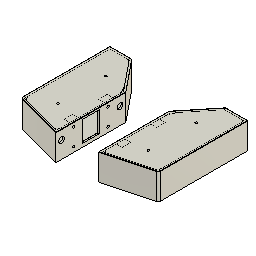
2_Assembly_Chassis v11 (Autodesk Fusion 360 archive; units mm, degrees)
design "Back Extention"
Autodesk Fusion 360 part; units mm, degrees
(part 1 of 2)
sketch "Sketch1" plane through (0, 0, 0) normal (0, 0, 1) x (1, 0, 0)
  line L0 (0, 0) -> (0, 121.8)
  line L1 (0, 0) -> (78.294095, 20.97884)
  line L2 (82, 25.808469) -> (82, 176.135475)
  line L3 (82, 176.135475) -> (44, 176.135475)
  line L4 (44, 176.135475) -> (0, 121.8)
  arc A0 (78.294095, 20.97884) -> (82, 25.808469) centre (77, 25.808469) ccw
  line L5 (3, 3.909676) -> (77.517638, 23.876617)
  arc A1 (77.517638, 23.876617) -> (79, 25.808469) centre (77, 25.808469) ccw
  line L6 (79, 25.808469) -> (79, 173.135475)
  line L7 (79, 173.135475) -> (45.430927, 173.135475)
  line L8 (45.430927, 173.135475) -> (3, 120.737644)
  line L9 (3, 3.909676) -> (3, 120.737644)
  line L10 (3, 91.254041) -> (79, 91.254041) construction
  line L11 (41, 167.663736) -> (41, 14.091745) construction
  circle A2 centre (41, 128.135475) radius 5
  circle A3 centre (41, 45) radius 5
  dimension "d3" = 121.8
  dimension "d4" = 75
  dimension "d5" = 141
  dimension "d6" = 82
  dimension "d7" = 75
  dimension "d8" = 38
  dimension "d9" = 5
  dimension "d64" = -3
  dimension "d86" = 10
  dimension "d87" = 45
  dimension "d88" = 10
  dimension "d89" = 45
  constraint coincident L0.start L1.start
  constraint vertical L0
  constraint parallel L0 L2
  constraint perpendicular L0 L3
  constraint tangent L2 A0
  constraint tangent L1 A0
  constraint perpendicular L6 L10
  constraint perpendicular L10 L11
  constraint coincident L11 A3.centre
  measures "d3" distance of L0.start L0.end
  measures "d4" angle of L0 L1
  measures "d5" angle of L0 L4
  measures "d6" distance of L0 L2
  measures "d7" angle of L0 L1
  measures "d9" radius of A0
  measures "d86" diameter of A2
  measures "d88" diameter of A3
  measures "d89" vertical distance of L0.start A3.centre
extrude "Extrude7" add sketch "Sketch1" along normal blind 3 contours L5 A1 L6 L7 L8 L9 | A2 | A3 picked at (67.925955, 108.535214) picked at (43.631771, 126.680026) picked at (42.542117, 43.337994) makes body 1
extrude "Extrude13" add sketch "Sketch1" along normal blind 45 contours L0 L1 L2 L3 L4 A0 | A2 | A3 picked at (81, 125.026473) picked at (43.631771, 126.680026) picked at (42.542117, 43.337994) bodies 1
sketch "Sketch2" plane through (0, 0, 0) normal (-1, 0, 0) x (0, -1, 0)
  line L0 (-121.8, 0) -> (0, 0)
  line L1 (0, 0) -> (0, 45)
  line L2 (0, 45) -> (-121.8, 45)
  line L3 (-121.8, 45) -> (-121.8, 0)
  line L4 (-45.9, 42) -> (-75.9, 42)
  line L5 (-75.9, 42) -> (-75.9, 6)
  line L6 (-75.9, 6) -> (-45.9, 6)
  line L7 (-45.9, 6) -> (-45.9, 42)
  line L8 (-45.9, 42) -> (-75.9, 6) construction
  line L9 (-75.9, 42) -> (-45.9, 6) construction
  line L10 (-60.9, 45) -> (-60.9, 0) construction
  line L11 (-30.9, 39) -> (-90.9, 39) construction
  line L12 (-90.9, 39) -> (-90.9, 9) construction
  line L13 (-90.9, 9) -> (-30.9, 9) construction
  line L14 (-30.9, 9) -> (-30.9, 39) construction
  line L15 (-30.9, 39) -> (-90.9, 9) construction
  line L16 (-90.9, 39) -> (-30.9, 9) construction
  circle A0 centre (-90.9, 9) radius 2.1
  circle A1 centre (-90.9, 39) radius 2.1
  circle A2 centre (-30.9, 9) radius 2.1
  circle A3 centre (-30.9, 39) radius 2.1
  line L17 (0, 29.417) -> (-121.8, 29.417) construction
  circle A4 centre (-10, 29.417) radius 5
  circle A5 centre (-111.8, 29.417) radius 5
  line L18 (-121.8, 0) -> (0, 0)
  line L19 (0, 0) -> (0, 45)
  line L20 (0, 45) -> (-121.8, 45)
  line L21 (-121.8, 45) -> (-121.8, 0)
  point P0 (-60.9, 24)
  point P1 (-60.9, 24)
  dimension "d16" = 30
  dimension "d17" = 36
  dimension "d19" = 60
  dimension "d20" = 30
  dimension "d21" = 4.2
  dimension "d22" = 4.2
  dimension "d23" = 4.2
  dimension "d24" = 4.2
  dimension "d26" = 50.9
  dimension "d27" = 10
  dimension "d54" = 30.9
  dimension "d55" = 90.9
  dimension "d67" = 29.417
  dimension "d68" = 6
  constraint horizontal L4
  constraint perpendicular L4 L5
  constraint parallel L4 L6
  constraint parallel L5 L7
  constraint coincident L8 P1
  constraint coincident L9 P1
  constraint midpoint L2 L10.start
  constraint midpoint L0 L10.end
  constraint coincident P1 L10
  constraint horizontal L11
  constraint perpendicular L11 L12
  constraint parallel L11 L13
  constraint parallel L12 L14
  constraint coincident L15 P1
  constraint coincident L16 P1
  constraint coincident P1 P0
  constraint coincident L12.end L13.start
  constraint coincident L11.end L12.start
  constraint coincident L13.end L14.start
  constraint coincident L11.start L14.end
  constraint coincident L1 L17.start
  constraint coincident L3 L17.end
  constraint perpendicular L3 L17
  constraint coincident L17 A4.centre
  constraint symmetric L10 A4 A5
  measures "d16" distance of L5.end L6.end
  measures "d17" distance of L4.end L5.end
  measures "d19" distance of L12.end L13.end
  measures "d20" distance of L11.end L12.end
  measures "d21" diameter of A0
  measures "d22" diameter of A1
  measures "d23" diameter of A2
  measures "d24" diameter of A3
  measures "d26" distance of L10 A4.centre
  measures "d27" diameter of A4
  measures "d54" horizontal distance of L0.end L13.end
  measures "d55" horizontal distance of L0.end L12.end
  measures "d67" distance of L0.end L17.start
  measures "d68" vertical distance of L0.end L6.end
extrude "Extrude16" cut sketch "Sketch2" against normal blind 10 contours L4 L5 L6 L7 | A0 | A1 | A2 | A3 | A4 | A5 picked at (-65.9, 18) picked at (-90.207818, 8.89567) picked at (-91.354622, 39.606218) picked at (-32.17464, 9.251722) picked at (-31.534769, 38.918203) picked at (-10.833333, 30.579729) picked at (-113.210608, 28.925741) bodies 1
sketch "Sketch3" plane through (0, 176.135475, 0) normal (0, 1, 0) x (-1, 0, 0)
  line L0 (-82, 0) -> (-44, 0)
  line L1 (-44, 0) -> (-44, 45)
  line L2 (-44, 45) -> (-82, 45)
  line L3 (-82, 45) -> (-82, 0)
  line L4 (-44, 45) -> (-82, 0) construction
  line L5 (-50.5, 7.5) -> (-75.5, 7.5) construction
  line L6 (-75.5, 7.5) -> (-75.5, 37.5) construction
  line L7 (-75.5, 37.5) -> (-50.5, 37.5) construction
  line L8 (-50.5, 37.5) -> (-50.5, 7.5) construction
  line L9 (-50.5, 7.5) -> (-75.5, 37.5) construction
  line L10 (-75.5, 7.5) -> (-50.5, 37.5) construction
  circle A0 centre (-75.5, 37.5) radius 1.6
  circle A1 centre (-50.5, 37.5) radius 1.6
  circle A2 centre (-75.5, 7.5) radius 1.6
  circle A3 centre (-50.5, 7.5) radius 1.6
  circle A4 centre (-63, 22.5) radius 12.5
  line L11 (-82, 0) -> (-44, 0)
  line L12 (-44, 0) -> (-44, 45)
  line L13 (-44, 45) -> (-82, 45)
  line L14 (-82, 45) -> (-82, 0)
  point P0 (-63, 22.5)
  dimension "d30" = 3.2
  dimension "d31" = 3.2
  dimension "d32" = 3.2
  dimension "d33" = 3.2
  dimension "d34" = 25
  dimension "d35" = 30
  dimension "d36" = 25
  constraint coincident L1.end L2.start
  constraint coincident L0.start L3.end
  constraint horizontal L5
  constraint perpendicular L5 L6
  constraint parallel L5 L7
  constraint parallel L6 L8
  constraint coincident L9 P0
  constraint coincident L10 P0
  constraint midpoint L4 P0
  constraint coincident L6.end L7.start
  constraint coincident L7.end L8.start
  constraint coincident L5.end L6.start
  constraint coincident L5.start L8.end
  constraint coincident P0 A4.centre
  measures "d30" diameter of A0
  measures "d31" diameter of A1
  measures "d32" diameter of A2
  measures "d33" diameter of A3
  measures "d34" distance of L6.end L7.end
  measures "d35" distance of L5.end L6.end
  measures "d36" diameter of A4
extrude "Extrude17" cut sketch "Sketch3" against normal blind 10 contours A0 | A1 | A2 | A3 | A4 picked at (-75.766667, 36.57531) picked at (-50.233333, 38.276286) picked at (-75.167472, 8.379786) picked at (-50.167472, 8.231382) picked at (-57.779901, 21.179037) bodies 1
sketch "Sketch5" plane through (0, 0, 45) normal (0, 0, 1) x (-1, 0, 0)
  circle A0 centre (-41, -45) radius 5
  circle A1 centre (-41, -128.135475) radius 5
  circle A2 centre (-41, -128.135475) radius 0.75
  circle A3 centre (-41, -45) radius 0.75
  circle A4 centre (-41, -45) radius 5
  dimension "d90" = 1.5
  dimension "d91" = 1.5
  constraint concentric A1 A2
  constraint concentric A0 A3
  measures "d90" diameter of A2
  measures "d91" diameter of A3
fillet "Fillet2" radius 2.5 6 edges at (3, 62.32366, 3) (24.215463, 146.93656, 3) (62.215463, 173.135475, 3) (40.258819, 13.893147, 3) (78.586707, 24.590946, 3) (79, 99.471972, 3) on bodies 1
fillet "Fillet2" radius 2.5 2 edges at (36.338363, 129.943552, 3) (36.338363, 46.808077, 3) on bodies 1
extrude "Extrude14" cut 2 faces at (42.542117, 43.337994, 45) (43.631771, 126.680026, 45) along direction (0, 0, -1) blind 3 on bodies 1 bodies 1
extrude "Extrude15" cut sketch "Sketch5" against normal blind 20 contours A2 | A3 picked at (-41.367375, -128.379207) picked at (-40.981317, -45.101923) bodies 1
sketch "Sketch4" plane through (0, 0, 45) normal (0, 0, 1) x (1, 0, 0)
  arc A0 (77.517638, 23.876617) -> (79, 25.808469) centre (77, 25.808469) ccw
  line L0 (77.517638, 23.876617) -> (3, 3.909676)
  line L1 (3, 3.909676) -> (3, 120.737644)
  line L2 (3, 120.737644) -> (45.430927, 173.135475)
  line L3 (45.430927, 173.135475) -> (79, 173.135475)
  line L4 (79, 173.135475) -> (79, 25.808469)
  line L5 (0, 0) -> (78.294095, 20.97884)
  arc A1 (78.294095, 20.97884) -> (82, 25.808469) centre (77, 25.808469) ccw
  line L6 (82, 25.808469) -> (82, 176.135475)
  line L7 (82, 176.135475) -> (44, 176.135475)
  line L8 (44, 176.135475) -> (0, 121.8)
  line L9 (0, 121.8) -> (0, 0)
  line L10 (3, 106.572901) -> (3, 10.425803)
  line L11 (11.914162, 131.745717) -> (42.429222, 169.428679)
  line L12 (50.200682, 173.135475) -> (74, 173.135475)
  line L13 (79, 168.135475) -> (79, 31.947085)
  line L14 (9.294095, 5.596174) -> (71.58819, 22.287826)
  arc A2 (11.914162, 131.745717) -> (3, 106.572901) centre (43, 106.572901) ccw
  arc A3 (50.200682, 173.135475) -> (42.429222, 169.428679) centre (50.200682, 163.135475) ccw
  arc A4 (79, 168.135475) -> (74, 173.135475) centre (74, 168.135475) ccw
  arc A5 (3, 10.425803) -> (9.294095, 5.596174) centre (8, 10.425803) ccw
  arc A6 (71.58819, 22.287826) -> (79, 31.947085) centre (69, 31.947085) ccw
  line L15 (13, 27.309676) -> (3, 27.309676)
  line L16 (3, 27.309676) -> (3, 42.309676)
  line L17 (3, 42.309676) -> (13, 42.309676)
  line L18 (13, 42.309676) -> (13, 27.309676)
  line L19 (13, 27.309676) -> (3, 42.309676) construction
  line L20 (3, 27.309676) -> (13, 42.309676) construction
  line L21 (13, 87.309676) -> (3, 87.309676)
  line L22 (3, 87.309676) -> (3, 102.309676)
  line L23 (3, 102.309676) -> (13, 102.309676)
  line L24 (13, 102.309676) -> (13, 87.309676)
  line L25 (13, 87.309676) -> (3, 102.309676) construction
  line L26 (3, 87.309676) -> (13, 102.309676) construction
  arc A7 (77.517638, 23.876617) -> (79, 25.808469) centre (77, 25.808469) ccw
  line L27 (77.517638, 23.876617) -> (3, 3.909676)
  line L28 (3, 3.909676) -> (3, 120.737644)
  line L29 (3, 120.737644) -> (45.430927, 173.135475)
  line L30 (45.430927, 173.135475) -> (79, 173.135475)
  line L31 (79, 173.135475) -> (79, 25.808469)
  line L32 (0, 0) -> (78.294095, 20.97884)
  arc A8 (78.294095, 20.97884) -> (82, 25.808469) centre (77, 25.808469) ccw
  line L33 (82, 25.808469) -> (82, 176.135475)
  line L34 (82, 176.135475) -> (44, 176.135475)
  line L35 (44, 176.135475) -> (0, 121.8)
  line L36 (0, 121.8) -> (0, 0)
  circle A9 centre (41, 128.135475) radius 0.75
  circle A10 centre (41, 45) radius 0.75
  circle A11 centre (41, 128.135475) radius 1.75
  circle A12 centre (41, 45) radius 1.75
  point P0 (8, 34.809676)
  point P1 (8, 94.809676)
  dimension "d69" = 40
  dimension "d70" = 10
  dimension "d71" = 5
  dimension "d72" = 5
  dimension "d73" = 10
  dimension "d74" = 10
  dimension "d75" = 15
  dimension "d76" = 10
  dimension "d77" = 15
  dimension "d78" = 30.9
  dimension "d79" = 90.9
  dimension "d108" = 3.5
  dimension "d109" = 3.5
  constraint tangent L11 A2
  constraint tangent L10 A2
  constraint tangent L11 A3
  constraint tangent L12 A3
  constraint tangent L12 A4
  constraint tangent L13 A4
  constraint tangent L10 A5
  constraint tangent L14 A5
  constraint tangent L14 A6
  constraint tangent L13 A6
  constraint horizontal L15
  constraint perpendicular L15 L16
  constraint parallel L15 L17
  constraint parallel L16 L18
  constraint horizontal L21
  constraint perpendicular L21 L22
  constraint parallel L21 L23
  constraint parallel L22 L24
  constraint concentric A9 A11
  constraint concentric A10 A12
  measures "d69" radius of A2
  measures "d70" radius of A3
  measures "d71" radius of A4
  measures "d72" radius of A5
  measures "d73" radius of A6
  measures "d108" diameter of A11
  measures "d109" diameter of A12
extrude "Extrude8" add sketch "Sketch4" against normal blind 3 separate body contours L0 L1 L2 L3 L4 L10 L11 L12 L13 L14 A2 A3 A4 A5 A6 L15 L17 L18 L21 L23 L24 L27 L28 L29 L30 L31 picked at (66.866235, 109.168748) makes body 2
extrude "Extrude10" add sketch "Sketch4" along normal blind 1 contours A0 L0 L4 A6 A7 L27 L31 | L0 L1 L2 L3 L4 L10 L11 L12 L13 L14 A2 A3 A4 A5 A6 L15 L17 L18 L21 L23 L24 L27 L28 L29 L30 L31 | L0 L1 A5 L27 L28 | L3 L4 A4 L30 L31 | L1 L10 L15 L16 L17 L18 L28 | L2 L3 A3 L29 L30 | L1 L10 L21 L22 L23 L24 L28 | L1 L2 A2 L28 L29 | L5 A1 L6 L7 L8 L9 L32 A8 L33 L34 L35 L36 picked at (77.498701, 25.486857) picked at (66.866235, 109.168748) picked at (4.309167, 5.615816) picked at (78.017684, 172.153159) picked at (6.333333, 37.309676) picked at (46.201154, 172.665108) picked at (6.333333, 97.309676) picked at (4.587771, 120.175385) picked at (1, 49.703225) bodies 2
mirror "Mirror3" about plane through (0, 0, 0) normal (1, 0, 0) of bodies 1 makes body 3
move_body "Move5" bodies 3 to x (1, 0, 0) y (0, 1, 0) z (0, 0, 1) at (-50, 0, 0)
mirror "Mirror4" about plane through (0, 0, 0) normal (1, 0, 0) of bodies 2 makes body 4
move_body "Move6" bodies 4 to x (1, 0, 0) y (0, 1, 0) z (0, 0, 1) at (-50, 0, 0)
copy_body "Body->Comp1" bodies 1 removing the originals makes body 5 in component "Back Ext - Right"
copy_body "Body->Comp2" bodies 2 removing the originals makes body 6 in component "Back Ext Cover - Right"
copy_body "Body->Comp3" bodies 3 removing the originals makes body 7 in component "Back Ext - Left"
copy_body "Body->Comp4" bodies 4 removing the originals makes body 8 in component "Back Ext Cover - Left"
component "Back Ext - Right" placed x (1, 0, 0) y (0, 1, 0) z (0, 0, 1) at (0, 0, 0)
component "Back Ext Cover - Right" placed x (1, 0, 0) y (0, 1, 0) z (0, 0, 1) at (0, 0, 0)
component "Back Ext - Left" placed x (1, 0, 0) y (0, 1, 0) z (0, 0, 1) at (0, 0, 0)
component "Back Ext Cover - Left" placed x (1, 0, 0) y (0, 1, 0) z (0, 0, 1) at (0, 0, 0)
equation "d26 = ( 101.8 / 2 ) * 1 mm"
named bodies: "Back2 - Right", "Back - Right", "Back - Left", "Back2 - Left"

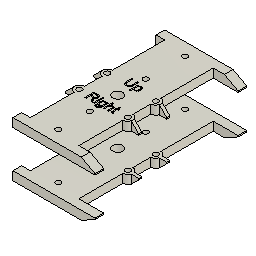
design "Support Suspension - OUT"
Autodesk Fusion 360 part; units mm, degrees
sketch "Sketch1" plane through (0, 0, 0) normal (0, 0, 1) x (1, 0, 0)
  line L0 (19.5, 61) -> (-19.5, 61)
  line L1 (-19.5, 61) -> (-19.5, -61)
  line L2 (-19.5, -61) -> (19.5, -61)
  line L3 (19.5, -61) -> (19.5, 61)
  line L4 (19.5, 61) -> (-19.5, -61) construction
  line L5 (-19.5, 61) -> (19.5, -61) construction
  line L6 (-26.5, 61) -> (39.5, 61)
  line L7 (39.5, 61) -> (39.5, 54)
  line L8 (39.5, 54) -> (-26.5, 54)
  line L9 (-26.5, 54) -> (-26.5, 61)
  line L10 (-19.5, 0) -> (19.5, 0) construction
  line L11 (39.5, -54) -> (-26.5, -54)
  line L12 (-26.5, -54) -> (-26.5, -61)
  line L13 (-26.5, -61) -> (39.5, -61)
  line L14 (39.5, -61) -> (39.5, -54)
  line L15 (-19.5, -3.3) -> (19.5, -3.3) construction
  line L16 (0, 0) -> (0, -64.5802) construction
  circle A0 centre (0, -3.3) radius 22.5 construction
  circle A1 centre (0, 19.2) radius 2.1
  circle A2 centre (-19.4856, 7.95) radius 2.1
  circle A3 centre (-19.4856, -14.55) radius 2.1
  circle A4 centre (0, -25.8) radius 2.1
  circle A5 centre (19.4856, -14.55) radius 2.1
  circle A6 centre (19.4856, 7.95) radius 2.1
  circle A7 centre (-19.4856, 7.95) radius 4
  circle A8 centre (-19.4856, -14.55) radius 4
  circle A9 centre (19.4856, 7.95) radius 4
  circle A10 centre (19.4856, -14.55) radius 4
  line L17 (19.4856, 6.7) -> (29.4856, 6.7)
  line L18 (29.4856, 6.7) -> (29.4856, 9.2)
  line L19 (29.4856, 9.2) -> (19.4856, 9.2)
  line L20 (19.4856, 9.2) -> (19.4856, 6.7)
  line L21 (0, 0) -> (0, 19.2) construction
  line L22 (29.4856, 9.2) -> (19.4856, 9.2)
  line L23 (19.4856, 9.2) -> (19.4856, 6.7)
  line L24 (19.4856, 6.7) -> (29.4856, 6.7)
  line L25 (29.4856, 6.7) -> (29.4856, 9.2)
  line L26 (29.4856, 9.2) -> (19.4856, 9.2)
  line L27 (19.4856, 9.2) -> (19.4856, 6.7)
  line L28 (19.4856, 6.7) -> (29.4856, 6.7)
  line L29 (29.4856, 6.7) -> (29.4856, 9.2)
  line L30 (29.4856, -13.3) -> (19.4856, -13.3)
  line L31 (19.4856, -13.3) -> (19.4856, -15.8)
  line L32 (19.4856, -15.8) -> (29.4856, -15.8)
  line L33 (29.4856, -15.8) -> (29.4856, -13.3)
  line L34 (-19.4856, 9.2) -> (-29.4856, 9.2)
  line L35 (-29.4856, 9.2) -> (-29.4856, 6.7)
  line L36 (-29.4856, 6.7) -> (-19.4856, 6.7)
  line L37 (-19.4856, 6.7) -> (-19.4856, 9.2)
  line L38 (-19.4856, -13.3) -> (-29.4856, -13.3)
  line L39 (-29.4856, -13.3) -> (-29.4856, -15.8)
  line L40 (-29.4856, -15.8) -> (-19.4856, -15.8)
  line L41 (-19.4856, -15.8) -> (-19.4856, -13.3)
  circle A11 centre (0, -3.3) radius 4
  circle A12 centre (0, 51) radius 2.1
  line L42 (0, 61) -> (0, -61) construction
  circle A13 centre (0, -51) radius 2.1
  dimension "d1" = 122
  dimension "d9" = 39
  dimension "d10" = 7
  dimension "d11" = 7
  dimension "d12" = 20
  dimension "d13" = 3.3
  dimension "d14" = 45
  dimension "d15" = 4.2
  dimension "d17" = 360
  dimension "d18" = 8
  dimension "d19" = 8
  dimension "d20" = 8
  dimension "d21" = 8
  dimension "d28" = 2.5
  dimension "d29" = 10
  dimension "d30" = 2.5
  dimension "d31" = 10
  dimension "d32" = 2.5
  dimension "d33" = 10
  dimension "d34" = 2.5
  dimension "d35" = 10
  dimension "d36" = 2.5
  dimension "d37" = 10
  dimension "d38" = 2.5
  dimension "d39" = 10
  dimension "d41" = 8
  dimension "d51" = 4.2
  dimension "d52" = 10
  dimension "d53" = 4.2
  dimension "d54" = 10
  constraint perpendicular L0 L1
  constraint parallel L0 L2
  constraint parallel L1 L3
  constraint horizontal L0
  constraint horizontal L6
  constraint vertical L7
  constraint horizontal L8
  constraint vertical L9
  constraint coincident L0.end L6
  constraint midpoint L1 L10.start
  constraint midpoint L3 L10.end
  constraint symmetric L6.start L10 L12.end
  constraint symmetric L6.end L10 L13.end
  constraint symmetric L7.end L10 L11.start
  constraint symmetric L8.end L10 L11.end
  constraint coincident L1 L15.start
  constraint coincident L3 L15.end
  constraint perpendicular L3 L15
  constraint coincident L16.start L21.start
  constraint perpendicular L11 L16
  constraint midpoint L15 A0.centre
  constraint coincident A0 A1.centre
  constraint concentric A2 A7
  constraint concentric A3 A8
  constraint concentric A6 A9
  constraint concentric A5 A10
  constraint horizontal L17
  constraint vertical L18
  constraint horizontal L19
  constraint vertical L20
  constraint midpoint A6.centre L20
  constraint coincident A1.centre L21.end
  constraint vertical L21
  constraint coincident L16.start L10
  constraint midpoint L16.start L10
  constraint horizontal L24
  constraint vertical L25
  constraint horizontal L22
  constraint vertical L23
  constraint horizontal L28
  constraint vertical L29
  constraint horizontal L26
  constraint vertical L27
  constraint horizontal L32
  constraint vertical L33
  constraint horizontal L30
  constraint vertical L31
  constraint midpoint A5.centre L31
  constraint horizontal L36
  constraint vertical L37
  constraint horizontal L34
  constraint vertical L35
  constraint midpoint A2.centre L37
  constraint horizontal L40
  constraint vertical L41
  constraint horizontal L38
  constraint vertical L39
  constraint midpoint A3.centre L41
  constraint concentric A0 A11
  constraint midpoint L0 L42.start
  constraint midpoint L2 L42.end
  constraint coincident A12.centre L42
  constraint coincident L16 A13.centre
  measures "d1" distance of L0.end L1.end
  measures "d9" distance of L0.start L0.end
  measures "d10" distance of L6.start L8.end
  measures "d11" distance of L0.end L6.start
  measures "d12" distance of L0.start L6.end
  measures "d13" distance of L10 L15
  measures "d14" diameter of A0
  measures "d15" diameter of A1
  measures "d18" diameter of A7
  measures "d19" diameter of A8
  measures "d20" diameter of A9
  measures "d21" diameter of A10
  measures "d28" distance of L17.end L18.end
  measures "d29" distance of L18.end L19.end
  measures "d30" distance of L17.end L18.end
  measures "d31" distance of L19.end L18.end
  measures "d32" distance of L17.end L18.end
  measures "d33" distance of L19.end L18.end
  measures "d34" distance of L32.end L30.start
  measures "d35" distance of L30.end L30.start
  measures "d36" distance of L36.end L34.start
  measures "d37" distance of L34.end L34.start
  measures "d38" distance of L40.end L38.start
  measures "d39" distance of L38.end L38.start
  measures "d41" diameter of A11
  measures "d51" diameter of A12
  measures "d52" distance of L6 A12.centre
  measures "d53" diameter of A13
  measures "d54" distance of L13 A13.centre
extrude "Extrude1" add sketch "Sketch1" along normal blind 7 contours L0 L1 L3 L6 L8 | L3 L6 L7 L8 | L1 L6 L8 L9 | L1 L3 L8 L11 A7 A8 A9 A10 | L3 A6 A9 L19 L22 L26 | L3 A6 A9 | L1 A2 A7 | L1 A2 A7 L34 | A9 L17 L18 L19 L22 L24 L25 L26 L28 L29 | A6 A9 L17 L19 L22 L24 L26 L28 | L3 A6 A9 L17 L24 L28 | A2 A7 L34 L36 | A7 L34 L35 L36 | L3 A5 A10 L30 | L3 A5 A10 | L1 A2 A7 L36 | A10 L30 L32 L33 | A5 A10 L30 L32 | L3 A5 A10 L32 | L1 A3 A8 | L1 A3 A8 L38 | L3 L11 L13 L14 | L1 L2 L3 L11 L13 | A3 A8 L38 L40 | A8 L38 L39 L40 | L1 L11 L12 L13 | L1 A3 A8 L40 makes body 1
chamfer "Chamfer1" distance 11 distance2 6 2 edges at (39.5, -57.5, 7) (39.5, 57.5, 7) measured on face at (-13.5784, 28.7776, 7) measured on face at (-13.5784, 28.7776, 7) on bodies 1
chamfer "Chamfer2" distance 6 angle 45 4 edges at (-29.4856, 7.95, 7) (-29.4856, -14.55, 7) (29.4856, 7.95, 7) (29.4856, -14.55, 7) on bodies 1
mirror "Mirror1" about plane through (0, 0, 0) normal (0, 0, 1) of bodies 1 makes body 2
sketch "Sketch3" plane through (0, 0, 7) normal (0, 0, 1) x (-1, 0, 0)
  line L0 (-23.4856, 15.8) -> (-23.4856, 13.3)
  line L1 (-23.4856, 13.3) -> (-23.2852, 13.3)
  arc A0 (-23.2852, 13.3) -> (-19.5, 10.55) centre (-19.4856, 14.55) ccw
  line L2 (-19.5, 10.55) -> (-19.5, -3.95)
  arc A1 (-19.5, -3.95) -> (-23.2852, -6.7) centre (-19.4856, -7.95) ccw
  line L3 (-23.2852, -6.7) -> (-23.4856, -6.7)
  line L4 (-23.4856, -6.7) -> (-23.4856, -9.2)
  line L5 (-23.4856, -9.2) -> (-23.2852, -9.2)
  arc A2 (-23.2852, -9.2) -> (-19.5, -11.95) centre (-19.4856, -7.95) ccw
  line L6 (-19.5, -11.95) -> (-19.5, -54)
  line L7 (-19.5, -54) -> (-28.5, -54)
  line L8 (-28.5, -54) -> (-28.5, -61)
  line L9 (-28.5, -61) -> (26.5, -61)
  line L10 (26.5, -61) -> (26.5, -54)
  line L11 (26.5, -54) -> (19.5, -54)
  line L12 (19.5, -54) -> (19.5, -11.95)
  arc A3 (19.5, -11.95) -> (23.2852, -9.2) centre (19.4856, -7.95) ccw
  line L13 (23.2852, -9.2) -> (23.4856, -9.2)
  line L14 (23.4856, -9.2) -> (23.4856, -6.7)
  line L15 (23.4856, -6.7) -> (23.2852, -6.7)
  arc A4 (23.2852, -6.7) -> (19.5, -3.95) centre (19.4856, -7.95) ccw
  line L16 (19.5, -3.95) -> (19.5, 10.55)
  arc A5 (19.5, 10.55) -> (23.2852, 13.3) centre (19.4856, 14.55) ccw
  line L17 (23.2852, 13.3) -> (23.4856, 13.3)
  line L18 (23.4856, 13.3) -> (23.4856, 15.8)
  line L19 (23.4856, 15.8) -> (23.2852, 15.8)
  arc A6 (23.2852, 15.8) -> (19.5, 18.55) centre (19.4856, 14.55) ccw
  line L20 (19.5, 18.55) -> (19.5, 54)
  line L21 (19.5, 54) -> (26.5, 54)
  line L22 (26.5, 54) -> (26.5, 61)
  line L23 (26.5, 61) -> (-28.5, 61)
  line L24 (-28.5, 61) -> (-28.5, 54)
  line L25 (-28.5, 54) -> (-19.5, 54)
  line L26 (-19.5, 54) -> (-19.5, 18.55)
  arc A7 (-19.5, 18.55) -> (-23.2852, 15.8) centre (-19.4856, 14.55) ccw
  line L27 (-23.2852, 15.8) -> (-23.4856, 15.8)
  circle A8 centre (0, -19.2) radius 2.1
  circle A9 centre (0, 25.8) radius 2.1
  circle A10 centre (0, 3.3) radius 4
  circle A11 centre (-19.4856, 14.55) radius 2.1
  circle A12 centre (-19.4856, -7.95) radius 2.1
  circle A13 centre (19.4856, -7.95) radius 2.1
  circle A14 centre (19.4856, 14.55) radius 2.1
  line L28 (11.6283, 20.1017) -> (-10.8571, 20.1017) construction
  line L29 (-10.8571, 20.1017) -> (-10.8571, 10.1017) construction
  line L30 (-10.8571, 10.1017) -> (11.6283, 10.1017) construction
  line L31 (11.6283, 10.1017) -> (11.6283, 20.1017) construction
  line L32 (6.0122, -4.7799) -> (-5.5845, -4.7799) construction
  line L33 (-5.5845, -4.7799) -> (-5.5845, -14.7799) construction
  line L34 (-5.5845, -14.7799) -> (6.0122, -14.7799) construction
  line L35 (6.0122, -14.7799) -> (6.0122, -4.7799) construction
  circle A15 centre (0, 51) radius 2.1
  circle A16 centre (0, -51) radius 2.1
  text T0 "Right" font "Arial" height 10 align ink ink in box 0 x 0 at (11.6283, 20.1017) x (-1, 0) y (0, -1) spacing 1 kerned height is em
  text T1 "Up" font "Arial" height 10 align ink ink in box 0 x 0 at (6.0122, -4.7799) x (-1, 0) y (0, -1) spacing 1 kerned height is em
  constraint perpendicular L28 L29
  constraint parallel L28 L30
  constraint parallel L29 L31
  constraint perpendicular L32 L33
  constraint parallel L32 L34
  constraint parallel L33 L35
extrude "Extrude3" cut sketch "Sketch3" against normal blind 1 text T0 T1 bodies 1
sketch "Sketch4" plane through (0, 0, -7) normal (0, 0, -1) x (1, 0, 0)
  circle A0 centre (-19.4856, 14.55) radius 2.1
  circle A1 centre (-19.4856, -7.95) radius 2.1
  circle A2 centre (19.4856, -7.95) radius 2.1
  circle A3 centre (19.4856, 14.55) radius 2.1
  circle A4 centre (0, 3.3) radius 4
  circle A5 centre (0, 25.8) radius 2.1
  circle A6 centre (0, -19.2) radius 2.1
  line L0 (23.4856, 13.3) -> (23.4856, 15.8)
  line L1 (23.4856, 15.8) -> (23.2852, 15.8)
  arc A7 (23.2852, 15.8) -> (19.5, 18.55) centre (19.4856, 14.55) ccw
  line L2 (19.5, 18.55) -> (19.5, 54)
  line L3 (19.5, 54) -> (28.5, 54)
  line L4 (28.5, 54) -> (28.5, 61)
  line L5 (28.5, 61) -> (-26.5, 61)
  line L6 (-26.5, 61) -> (-26.5, 54)
  line L7 (-26.5, 54) -> (-19.5, 54)
  line L8 (-19.5, 54) -> (-19.5, 18.55)
  arc A8 (-19.5, 18.55) -> (-23.2852, 15.8) centre (-19.4856, 14.55) ccw
  line L9 (-23.2852, 15.8) -> (-23.4856, 15.8)
  line L10 (-23.4856, 15.8) -> (-23.4856, 13.3)
  line L11 (-23.4856, 13.3) -> (-23.2852, 13.3)
  arc A9 (-23.2852, 13.3) -> (-19.5, 10.55) centre (-19.4856, 14.55) ccw
  line L12 (-19.5, 10.55) -> (-19.5, -3.95)
  arc A10 (-19.5, -3.95) -> (-23.2852, -6.7) centre (-19.4856, -7.95) ccw
  line L13 (-23.2852, -6.7) -> (-23.4856, -6.7)
  line L14 (-23.4856, -6.7) -> (-23.4856, -9.2)
  line L15 (-23.4856, -9.2) -> (-23.2852, -9.2)
  arc A11 (-23.2852, -9.2) -> (-19.5, -11.95) centre (-19.4856, -7.95) ccw
  line L16 (-19.5, -11.95) -> (-19.5, -54)
  line L17 (-19.5, -54) -> (-26.5, -54)
  line L18 (-26.5, -54) -> (-26.5, -61)
  line L19 (-26.5, -61) -> (28.5, -61)
  line L20 (28.5, -61) -> (28.5, -54)
  line L21 (28.5, -54) -> (19.5, -54)
  line L22 (19.5, -54) -> (19.5, -11.95)
  arc A12 (19.5, -11.95) -> (23.2852, -9.2) centre (19.4856, -7.95) ccw
  line L23 (23.2852, -9.2) -> (23.4856, -9.2)
  line L24 (23.4856, -9.2) -> (23.4856, -6.7)
  line L25 (23.4856, -6.7) -> (23.2852, -6.7)
  arc A13 (23.2852, -6.7) -> (19.5, -3.95) centre (19.4856, -7.95) ccw
  line L26 (19.5, -3.95) -> (19.5, 10.55)
  arc A14 (19.5, 10.55) -> (23.2852, 13.3) centre (19.4856, 14.55) ccw
  line L27 (23.2852, 13.3) -> (23.4856, 13.3)
  line L28 (6.1305, -3.1229) -> (-5.4662, -3.1229) construction
  line L29 (-5.4662, -3.1229) -> (-5.4662, -13.1229) construction
  line L30 (-5.4662, -13.1229) -> (6.1305, -13.1229) construction
  line L31 (6.1305, -13.1229) -> (6.1305, -3.1229) construction
  line L32 (8.3078, 18.4645) -> (-7.5662, 18.4645) construction
  line L33 (-7.5662, 18.4645) -> (-7.5662, 8.4645) construction
  line L34 (-7.5662, 8.4645) -> (8.3078, 8.4645) construction
  line L35 (8.3078, 8.4645) -> (8.3078, 18.4645) construction
  circle A15 centre (0, 51) radius 2.1
  circle A16 centre (0, -51) radius 2.1
  text T0 "Up" font "Arial" height 10 align ink ink in box 0 x 0 at (6.1305, -3.1229) x (-1, 0) y (0, -1) spacing 1 kerned height is em
  text T1 "Left" font "Arial" height 10 align ink ink in box 0 x 0 at (8.3078, 18.4645) x (-1, 0) y (0, -1) spacing 1 kerned height is em
  constraint perpendicular L28 L29
  constraint parallel L28 L30
  constraint parallel L29 L31
  constraint perpendicular L32 L33
  constraint parallel L32 L34
  constraint parallel L33 L35
extrude "Extrude5" cut sketch "Sketch4" against normal blind 1 text T0 T1 bodies 2
move_body "Move1" bodies 2 to x (1, 0, 0) y (0, 1, 0) z (0, 0, 1) at (0, 0, -30)
copy_body "Body->Comp1" bodies 1 removing the originals makes body 3 in component "Right"
copy_body "Body->Comp2" bodies 2 removing the originals makes body 4 in component "Left"
component "Right" placed x (1, 0, 0) y (0, 1, 0) z (0, 0, 1) at (0, 0, 0)
component "Left" placed x (1, 0, 0) y (0, 1, 0) z (0, 0, 1) at (0, 0, 0)
named bodies: "Right", "Left"

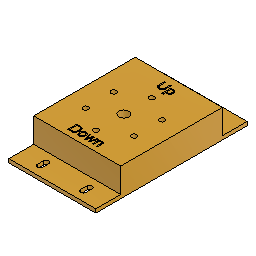
design "Support Suspension - IN"
Autodesk Fusion 360 part; units mm, degrees
sketch "Sketch1" plane through (0, 0, 0) normal (0, 0, 1) x (1, 0, 0)
  line L0 (-35, 60.9) -> (35, 60.9)
  line L1 (35, 60.9) -> (35, -60.9)
  line L2 (35, -60.9) -> (-35, -60.9)
  line L3 (-35, -60.9) -> (-35, 60.9)
  line L4 (-35, 60.9) -> (35, -60.9) construction
  line L5 (35, 60.9) -> (-35, -60.9) construction
  line L6 (35, -40.9) -> (-35, -40.9)
  line L7 (-35, -40.9) -> (-35, 40.9)
  line L8 (-35, 40.9) -> (35, 40.9)
  line L9 (35, 40.9) -> (35, -40.9)
  line L10 (35, -40.9) -> (-35, 40.9) construction
  line L11 (-35, -40.9) -> (35, 40.9) construction
  line L12 (-35, -3.3) -> (35, -3.3) construction
  circle A0 centre (0, -3.3) radius 4
  circle A1 centre (0, -3.3) radius 22.5 construction
  line L13 (0, 0) -> (0, 2.2401)
  line L14 (0, 2.2401) -> (0, 60.9) construction
  circle A2 centre (0, 19.2) radius 2.1
  circle A3 centre (-19.4856, 7.95) radius 2.1
  circle A4 centre (-19.4856, -14.55) radius 2.1
  circle A5 centre (0, -25.8) radius 2.1
  circle A6 centre (19.4856, -14.55) radius 2.1
  circle A7 centre (19.4856, 7.95) radius 2.1
  line L15 (-35, 60.9) -> (35, 40.9) construction
  line L16 (0, 50.9) -> (-35, 50.9) construction
  line L17 (0, 50.9) -> (35, 50.9) construction
  line L18 (-19.6, 53.4) -> (-19.6, 48.4)
  arc A8 (-19.6, 48.4) -> (-15.4, 48.4) centre (-17.5, 48.4) ccw
  line L19 (-15.4, 48.4) -> (-15.4, 53.4)
  arc A9 (-15.4, 53.4) -> (-19.6, 53.4) centre (-17.5, 53.4) ccw
  line L20 (-17.5, 53.4) -> (-17.5, 48.4) construction
  arc A10 (19.6, 53.4) -> (15.4, 53.4) centre (17.5, 53.4) ccw
  line L21 (19.6, 53.4) -> (19.6, 48.4)
  arc A11 (15.4, 48.4) -> (19.6, 48.4) centre (17.5, 48.4) ccw
  line L22 (15.4, 48.4) -> (15.4, 53.4)
  line L23 (-35, 0) -> (35, 0) construction
  arc A12 (15.4, -53.4) -> (19.6, -53.4) centre (17.5, -53.4) ccw
  arc A13 (-15.4, -48.4) -> (-19.6, -48.4) centre (-17.5, -48.4) ccw
  arc A14 (-19.6, -53.4) -> (-15.4, -53.4) centre (-17.5, -53.4) ccw
  arc A15 (19.6, -48.4) -> (15.4, -48.4) centre (17.5, -48.4) ccw
  line L24 (-17.5, -53.4) -> (-17.5, -48.4) construction
  line L25 (-15.4, -48.4) -> (-15.4, -53.4)
  line L26 (19.6, -53.4) -> (19.6, -48.4)
  line L27 (15.4, -48.4) -> (15.4, -53.4)
  line L28 (-19.6, -53.4) -> (-19.6, -48.4)
  line L29 (0, -50.9) -> (-35, -50.9) construction
  point P0 (-17.5, 50.9)
  point P1 (-17.5, -50.9)
  dimension "d1" = 121.8
  dimension "d2" = 70
  dimension "d3" = 81.8
  dimension "d4" = 44.2
  dimension "d5" = 38.6
  dimension "d6" = 8
  dimension "d7" = 45
  dimension "d8" = 4.2
  dimension "d10" = 360
  dimension "d13" = 4.2
  dimension "d14" = 5
  dimension "d19" = 3.3
  constraint perpendicular L0 L1
  constraint parallel L0 L2
  constraint parallel L1 L3
  constraint horizontal L0
  constraint coincident L4 L13.start
  constraint coincident L5 L13.start
  constraint coincident L13.start origin
  constraint perpendicular L6 L7
  constraint parallel L6 L8
  constraint parallel L7 L9
  constraint horizontal L6
  constraint coincident L1 L6.start
  constraint coincident L10 L13.start
  constraint coincident L11 L13.start
  constraint coincident L7 L12.start
  constraint coincident L9 L12.end
  constraint perpendicular L7 L12
  constraint midpoint L12 A0.centre
  constraint concentric A0 A1
  constraint vertical L13
  constraint midpoint L0 L14.end
  constraint coincident A1 A2.centre
  constraint coincident L14 A2.centre
  constraint midpoint L15 L16.start
  constraint coincident L3 L16.end
  constraint perpendicular L3 L16
  constraint coincident L1 L17.end
  constraint perpendicular L1 L17
  constraint tangent L18 A8
  constraint tangent A8 L19
  constraint parallel L18 L19
  constraint tangent L19 A9
  constraint tangent L18 A9
  constraint perpendicular L16 L20
  constraint midpoint L16 P0
  constraint midpoint L20 P0
  constraint symmetric L14 L18.start A10.start
  constraint symmetric L14 L18.end L21.end
  constraint symmetric L14 A8.end A11.start
  constraint symmetric L14 L19.end A10.end
  constraint symmetric L14 A8 A11
  constraint symmetric L14 A9 A10
  constraint midpoint L9 L23.end
  constraint perpendicular L9 L23
  constraint symmetric L16.start L23 L29.start
  constraint symmetric L16.end L23 L29.end
  constraint symmetric L18.start L23 A14.start
  constraint symmetric L18.end L23 A13.end
  constraint symmetric A8.end L23 A13.start
  constraint symmetric L19.end L23 A14.end
  constraint symmetric A8 L23 A13
  constraint symmetric A9 L23 A14
  constraint symmetric P0 L23 P1
  constraint symmetric A10.end L23 A12.start
  constraint symmetric A10.start L23 A12.end
  constraint symmetric A10 L23 A12
  constraint symmetric L21.end L23 A15.start
  constraint symmetric A11.start L23 A15.end
  constraint symmetric A11 L23 A15
  measures "d1" distance of L0.start L2.end
  measures "d2" distance of L0.start L0.end
  measures "d3" distance of L6.end L7.end
  measures "d4" distance of L8 L12
  measures "d6" diameter of A0
  measures "d7" diameter of A1 L0.start
  measures "d8" diameter of A2
  measures "d13" diameter of A8
  measures "d14" distance of A9.centre A8.centre
  measures "d19" distance of L13.start A0.centre
extrude "Extrude1" add sketch "Sketch1" along normal blind 19.8 contours L1 L3 L6 L7 L8 L9
extrude "Extrude2" add sketch "Sketch1" against normal blind 3
sketch "Sketch2" plane through (0, 0, 19.8) normal (0, 0, 1) x (-1, 0, 0)
  circle A0 centre (-19.4856, -7.95) radius 2.1
  circle A1 centre (-19.4856, 14.55) radius 2.1
  circle A2 centre (0, 25.8) radius 2.1
  circle A3 centre (19.4856, 14.55) radius 2.1
  circle A4 centre (19.4856, -7.95) radius 2.1
  circle A5 centre (0, -19.2) radius 2.1
  circle A6 centre (0, 3.3) radius 4
  line L0 (-35, -40.9) -> (35, -40.9)
  line L1 (35, -40.9) -> (35, 40.9)
  line L2 (35, 40.9) -> (-35, 40.9)
  line L3 (-35, 40.9) -> (-35, -40.9)
  line L4 (6.2801, -26.4921) -> (-5.3166, -26.4921) construction
  line L5 (-5.3166, -26.4921) -> (-5.3166, -36.4921) construction
  line L6 (-5.3166, -36.4921) -> (6.2801, -36.4921) construction
  line L7 (6.2801, -36.4921) -> (6.2801, -26.4921) construction
  line L8 (11.9175, 36.5887) -> (-12.1889, 36.5887) construction
  line L9 (-12.1889, 36.5887) -> (-12.1889, 26.5887) construction
  line L10 (-12.1889, 26.5887) -> (11.9175, 26.5887) construction
  line L11 (11.9175, 26.5887) -> (11.9175, 36.5887) construction
  text T0 "Up" font "Arial" height 10 align ink ink in box 0 x 0 at (6.2801, -26.4921) x (-1, 0) y (0, -1) spacing 1 kerned height is em
  text T1 "Down" font "Arial" height 10 align ink ink in box 0 x 0 at (11.9175, 36.5887) x (-1, 0) y (0, -1) spacing 1 kerned height is em
  constraint perpendicular L4 L5
  constraint parallel L4 L6
  constraint parallel L5 L7
  constraint perpendicular L8 L9
  constraint parallel L8 L10
  constraint parallel L9 L11
extrude "Extrude3" cut sketch "Sketch2" against normal blind 1 text T1 T0
named bodies: "Support Suspension"

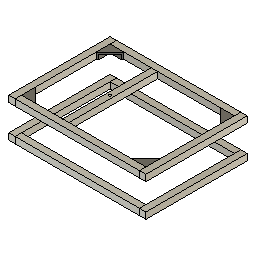
design "Aluminium Profiles 20x20"
Autodesk Fusion 360 part; units mm, degrees
sketch "Sketch1" plane through (0, 0, 0) normal (0, 1, 0) x (1, 0, 0)
  line L0 (10, 10) -> (-10, 10)
  line L1 (-10, 10) -> (-10, -10)
  line L2 (-10, -10) -> (10, -10)
  line L3 (10, -10) -> (10, 10)
  line L4 (10, 10) -> (-10, -10) construction
  line L5 (-10, 10) -> (10, -10) construction
  line L6 (20, 10) -> (20, -10)
  line L7 (20, -10) -> (40, -10)
  line L8 (40, -10) -> (40, 10)
  line L9 (40, 10) -> (20, 10)
  line L10 (50, 10) -> (50, -10)
  line L11 (50, -10) -> (70, -10)
  line L12 (70, -10) -> (70, 10)
  line L13 (70, 10) -> (50, 10)
  line L14 (100, 10) -> (80, 10)
  line L15 (80, 10) -> (80, -10)
  line L16 (80, -10) -> (100, -10)
  line L17 (100, -10) -> (100, 10)
  dimension "d1" = 20
  dimension "d2" = 20
  dimension "d5" = 20
  dimension "d6" = 20
  dimension "d9" = 20
  dimension "d10" = 20
  dimension "d145" = 20
  dimension "d146" = 20
  constraint perpendicular L0 L1
  constraint parallel L0 L2
  constraint parallel L1 L3
  constraint horizontal L0
  constraint coincident L4 origin
  constraint coincident L5 origin
  constraint perpendicular L6 L9
  constraint parallel L7 L9
  constraint parallel L6 L8
  constraint horizontal L9
  constraint perpendicular L10 L13
  constraint parallel L11 L13
  constraint parallel L10 L12
  constraint horizontal L13
  constraint perpendicular L14 L15
  constraint parallel L14 L16
  constraint parallel L15 L17
  constraint horizontal L14
  measures "d1" distance of L0.end L1.end
  measures "d2" distance of L1.end L2.end
  measures "d5" distance of L6.end L6.start
  measures "d6" distance of L7.end L6.end
  measures "d9" distance of L10.start L10.end
  measures "d10" distance of L11.end L10.end
  measures "d145" distance of L14.end L15.end
  measures "d146" distance of L16.end L15.end
extrude "Extrude1" add sketch "Sketch1" along normal blind 317 contours L0 L1 L2 L3 makes body 1
extrude "Extrude2" add sketch "Sketch1" along normal blind 389 separate body contours L6 L7 L8 L9 makes body 2
extrude "Extrude3" add sketch "Sketch1" along normal blind 82 separate body contours L10 L11 L12 L13 makes body 3
extrude "Extrude4" add sketch "Sketch1" along normal blind 277 separate body contours L14 L15 L16 L17 makes body 4
sketch "Sketch2" plane through (0, 0, 10) normal (0, 0, 1) x (-1, 0, 0)
  line L0 (-80, 0) -> (-100, 0)
  line L1 (-100, 0) -> (-100, -277)
  line L2 (-100, -277) -> (-80, -277)
  line L3 (-80, -277) -> (-80, 0)
  line L4 (-100, -277) -> (-80, 0) construction
  circle A0 centre (-90, -138.5) radius 4.1
  dimension "d149" = 8.2
  constraint coincident L1.end L2.start
  constraint coincident L0.start L3.end
  constraint midpoint L4 A0.centre
  measures "d149" diameter of A0
extrude "Extrude5" cut sketch "Sketch2" against normal through all contours A0 bodies 4
copy_body "Body->Comp1" bodies 3 removing the originals makes body 5 in component "Profile_20x20x82"
copy_body "Body->Comp2" bodies 1 removing the originals makes body 6 in component "Profile_20x20x317"
copy_body "Body->Comp3" bodies 2 removing the originals makes body 7 in component "Profile_20x20x389"
copy_body "Body->Comp4" bodies 4 removing the originals makes body 8 in component "Profile_20x20x277"
sketch "Sketch1 (2)" plane through (0, 0, 0) normal (0, 0, 1) x (1, 0, 0) in component "Corner Structure v3"
  line L0 (0, 0) -> (-45, 0)
  line L1 (0, 0) -> (0, 45)
  line L2 (0, 45) -> (-45, 0)
  line L3 (-5, 40) -> (-5, 5)
  line L4 (-5, 5) -> (-40, 5)
  line L5 (-2, 43) -> (0, 43)
  line L6 (-43, 2) -> (-43, 0)
  dimension "d1_1" = 45
  dimension "d2_1" = 45
  dimension "d5_1" = 5
  dimension "d6_1" = 5
  dimension "d7_1" = 2
  dimension "d8_1" = 2
  constraint coincident L0.start L1.start
  constraint horizontal L0
  constraint perpendicular L0 L1
  constraint coincident L2 L3.start
  constraint parallel L1 L3
  constraint coincident L2 L4.end
  constraint perpendicular L3 L4
  constraint coincident L2 L5.start
  constraint coincident L1 L5.end
  constraint perpendicular L1 L5
  constraint coincident L2 L6.start
  constraint coincident L0 L6.end
  constraint perpendicular L0 L6
  measures "d1_1" distance of L0.start L0.end
  measures "d2_1" distance of L0.start L1.end
  measures "d5_1" vertical distance of L0.start L3.end
  measures "d6_1" horizontal distance of L0.start L3.end
  measures "d7_1" distance of L0.end L6.end
  measures "d8_1" distance of L1.end L5.end
extrude "Extrude2'" add sketch "Sketch1 (2)" along normal blind 20 separate body contours L0 L1 L2 L3 L4 L5 L6 makes body 9 in component "Corner Structure v3"
extrude "Extrude3'" add sketch "Sketch1 (2)" along normal blind 5 contours L2 L3 L4 bodies 9 in component "Corner Structure v3"
sketch "Sketch1 (3)" plane through (0, 0, 0) normal (0, 0, 1) x (1, 0, 0) in component "Corner Structure v3 (1)"
  line L0 (0, 0) -> (-45, 0)
  line L1 (0, 0) -> (0, 45)
  line L2 (0, 45) -> (-45, 0)
  line L3 (-5, 40) -> (-5, 5)
  line L4 (-5, 5) -> (-40, 5)
  line L5 (-2, 43) -> (0, 43)
  line L6 (-43, 2) -> (-43, 0)
  dimension "d1_2" = 45
  dimension "d2_2" = 45
  dimension "d5_2" = 5
  dimension "d6_2" = 5
  dimension "d7_2" = 2
  dimension "d8_2" = 2
  constraint coincident L0.start L1.start
  constraint horizontal L0
  constraint perpendicular L0 L1
  constraint coincident L2 L3.start
  constraint parallel L1 L3
  constraint coincident L2 L4.end
  constraint perpendicular L3 L4
  constraint coincident L2 L5.start
  constraint coincident L1 L5.end
  constraint perpendicular L1 L5
  constraint coincident L2 L6.start
  constraint coincident L0 L6.end
  constraint perpendicular L0 L6
  measures "d1_2" distance of L0.start L0.end
  measures "d2_2" distance of L0.start L1.end
  measures "d5_2" vertical distance of L0.start L3.end
  measures "d6_2" horizontal distance of L0.start L3.end
  measures "d7_2" distance of L0.end L6.end
  measures "d8_2" distance of L1.end L5.end
extrude "Extrude2''" add sketch "Sketch1 (3)" along normal blind 20 separate body contours L0 L1 L2 L3 L4 L5 L6 makes body 10 in component "Corner Structure v3 (1)"
extrude "Extrude3''" add sketch "Sketch1 (3)" along normal blind 5 contours L2 L3 L4 bodies 10 in component "Corner Structure v3 (1)"
sketch "Sketch1 (4)" plane through (0, 0, 0) normal (0, 0, 1) x (1, 0, 0) in component "Corner Structure v3 (2)"
  line L0 (0, 0) -> (-45, 0)
  line L1 (0, 0) -> (0, 45)
  line L2 (0, 45) -> (-45, 0)
  line L3 (-5, 40) -> (-5, 5)
  line L4 (-5, 5) -> (-40, 5)
  line L5 (-2, 43) -> (0, 43)
  line L6 (-43, 2) -> (-43, 0)
  dimension "d1_3" = 45
  dimension "d2_3" = 45
  dimension "d5_3" = 5
  dimension "d6_3" = 5
  dimension "d7_3" = 2
  dimension "d8_3" = 2
  constraint coincident L0.start L1.start
  constraint horizontal L0
  constraint perpendicular L0 L1
  constraint coincident L2 L3.start
  constraint parallel L1 L3
  constraint coincident L2 L4.end
  constraint perpendicular L3 L4
  constraint coincident L2 L5.start
  constraint coincident L1 L5.end
  constraint perpendicular L1 L5
  constraint coincident L2 L6.start
  constraint coincident L0 L6.end
  constraint perpendicular L0 L6
  measures "d1_3" distance of L0.start L0.end
  measures "d2_3" distance of L0.start L1.end
  measures "d5_3" vertical distance of L0.start L3.end
  measures "d6_3" horizontal distance of L0.start L3.end
  measures "d7_3" distance of L0.end L6.end
  measures "d8_3" distance of L1.end L5.end
extrude "Extrude2'''" add sketch "Sketch1 (4)" along normal blind 20 separate body contours L0 L1 L2 L3 L4 L5 L6 makes body 11 in component "Corner Structure v3 (2)"
extrude "Extrude3'''" add sketch "Sketch1 (4)" along normal blind 5 contours L2 L3 L4 bodies 11 in component "Corner Structure v3 (2)"
sketch "Sketch1 (5)" plane through (0, 0, 0) normal (0, 0, 1) x (1, 0, 0) in component "Corner Structure v3 (3)"
  line L0 (0, 0) -> (-45, 0)
  line L1 (0, 0) -> (0, 45)
  line L2 (0, 45) -> (-45, 0)
  line L3 (-5, 40) -> (-5, 5)
  line L4 (-5, 5) -> (-40, 5)
  line L5 (-2, 43) -> (0, 43)
  line L6 (-43, 2) -> (-43, 0)
  dimension "d1_4" = 45
  dimension "d2_4" = 45
  dimension "d5_4" = 5
  dimension "d6_4" = 5
  dimension "d7_4" = 2
  dimension "d8_4" = 2
  constraint coincident L0.start L1.start
  constraint horizontal L0
  constraint perpendicular L0 L1
  constraint coincident L2 L3.start
  constraint parallel L1 L3
  constraint coincident L2 L4.end
  constraint perpendicular L3 L4
  constraint coincident L2 L5.start
  constraint coincident L1 L5.end
  constraint perpendicular L1 L5
  constraint coincident L2 L6.start
  constraint coincident L0 L6.end
  constraint perpendicular L0 L6
  measures "d1_4" distance of L0.start L0.end
  measures "d2_4" distance of L0.start L1.end
  measures "d5_4" vertical distance of L0.start L3.end
  measures "d6_4" horizontal distance of L0.start L3.end
  measures "d7_4" distance of L0.end L6.end
  measures "d8_4" distance of L1.end L5.end
extrude "Extrude2''''" add sketch "Sketch1 (5)" along normal blind 20 separate body contours L0 L1 L2 L3 L4 L5 L6 makes body 12 in component "Corner Structure v3 (3)"
extrude "Extrude3''''" add sketch "Sketch1 (5)" along normal blind 5 contours L2 L3 L4 bodies 12 in component "Corner Structure v3 (3)"
component "Profile_20x20x82" placed x (1, 0, 0) y (0, 0, 1) z (0, -1, 0) at (-88.5214, -13.0886, 13.8372)
component "Profile_20x20x317" placed x (1, 0, 0) y (0, 1, 0) z (0, 0, 1) at (-28.5214, -23.0886, 3.8372)
component "Profile_20x20x389" placed x (0, 1, 0) y (-1, 0, 0) z (0, 0, 1) at (370.4786, -43.0886, 3.8372)
component "Profile_20x20x277" placed x (1, 0, 0) y (0, 1, 0) z (0, 0, 1) at (29.9786, -3.0886, 105.8372)
component "Profile_20x20x317" placed x (-1, 0, 0) y (0, -1, 0) z (0, 0, 1) at (380.4786, 293.9114, 3.8372)
component "Profile_20x20x389" placed x (0, 1, 0) y (-1, 0, 0) z (0, 0, 1) at (370.4786, 253.9114, 3.8372)
component "Profile_20x20x317" placed x (1, 0, 0) y (0, 1, 0) z (0, 0, 1) at (-28.5214, -23.0886, 105.8372)
component "Profile_20x20x389" placed x (0, 1, 0) y (-1, 0, 0) z (0, 0, 1) at (370.4786, -43.0886, 105.8372)
component "Profile_20x20x317" placed x (-1, 0, 0) y (0, -1, 0) z (0, 0, 1) at (380.4786, 293.9114, 105.8372)
component "Profile_20x20x389" placed x (0, 1, 0) y (-1, 0, 0) z (0, 0, 1) at (370.4786, 253.9114, 105.8372)
component "Profile_20x20x82" placed x (1, 0, 0) y (0, 0, 1) z (0, -1, 0) at (320.4786, -13.0886, 13.8372)
component "Profile_20x20x82" placed x (1, 0, 0) y (0, 0, 1) z (0, -1, 0) at (320.4786, 283.9114, 13.8372)
component "Profile_20x20x82" placed x (1, 0, 0) y (0, 0, 1) z (0, -1, 0) at (-88.5214, 283.9114, 13.8372)
component "Corner Structure v3" placed x (0, 1, 0) y (1, 0, 0) z (0, 0, -1) at (-18.5214, 273.9114, 115.8372)
component "Corner Structure v3 (1)" placed x (-1, 0, 0) y (0, 1, 0) z (0, 0, -1) at (-18.5214, -3.0886, 115.8372)
component "Corner Structure v3 (2)" placed x (1, 0, 0) y (0, -1, 0) z (0, 0, -1) at (370.4786, 273.9114, 115.8372)
component "Corner Structure v3 (3)" placed x (0, -1, 0) y (-1, 0, 0) z (0, 0, -1) at (370.4786, -3.0886, 115.8372)
named bodies: "Profil20x20_317", "Profil20x20_389", "Profil20x20_82", "Profil20x20_277"

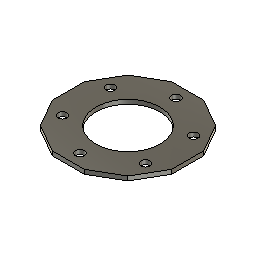
design "Rondelle suspension"
Autodesk Fusion 360 part; units mm, degrees
sketch "Sketch1" plane through (0, 0, 0) normal (0, 0, 1) x (1, 0, 0)
  line L0 (-7.5026, 28) -> (-20.4974, 20.4974)
  line L1 (-20.4974, 20.4974) -> (-28, 7.5026)
  line L2 (-28, 7.5026) -> (-28, -7.5026)
  line L3 (-28, -7.5026) -> (-20.4974, -20.4974)
  line L4 (-20.4974, -20.4974) -> (-7.5026, -28)
  line L5 (-7.5026, -28) -> (7.5026, -28)
  line L6 (7.5026, -28) -> (20.4974, -20.4974)
  line L7 (20.4974, -20.4974) -> (28, -7.5026)
  line L8 (28, -7.5026) -> (28, 7.5026)
  line L9 (28, 7.5026) -> (20.4974, 20.4974)
  line L10 (20.4974, 20.4974) -> (7.5026, 28)
  line L11 (7.5026, 28) -> (-7.5026, 28)
  circle A0 centre (0, 0) radius 22.5 construction
  line L12 (0, 0) -> (0, 28) construction
  circle A1 centre (0, 22.5) radius 2.1
  circle A2 centre (-19.4856, 11.25) radius 2.1
  circle A3 centre (-19.4856, -11.25) radius 2.1
  circle A4 centre (0, -22.5) radius 2.1
  circle A5 centre (19.4856, -11.25) radius 2.1
  circle A6 centre (19.4856, 11.25) radius 2.1
  circle A7 centre (0, 0) radius 15
  dimension "d1" = 28
  dimension "d2" = 45
  dimension "d3" = 4.2
  dimension "d5" = 360
  dimension "d6" = 30
  constraint coincident A0.centre L12.start
  constraint midpoint L11 L12.end
  constraint coincident A0 A1.centre
  constraint coincident L12 A1.centre
  constraint concentric A0 A7
  measures "d1" distance of A0.centre L11
  measures "d2" diameter of A0
  measures "d3" diameter of A1
  measures "d6" diameter of A7
extrude "Extrude1" add sketch "Sketch1" along normal blind 2

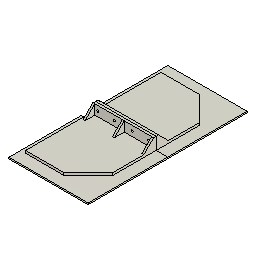
design "Up Cover"
Autodesk Fusion 360 part; units mm, degrees